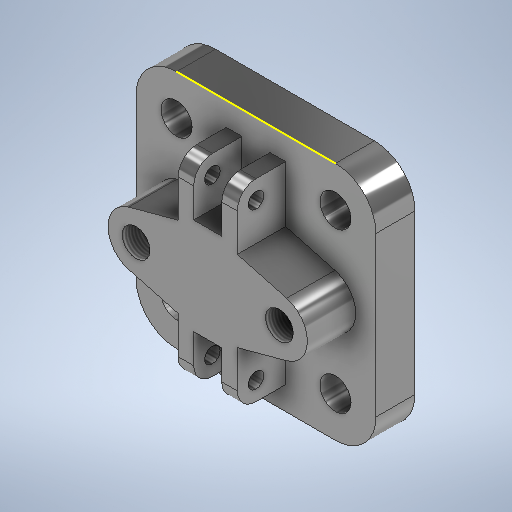
# Autodesk Inventor part: cad@74
Saved by Autodesk Inventor 2025.2 (Build 292293000, 293)
## iProperties
Created: 2025-04-27
Part Number: cad@74
Material: Generic
Document SubType Name: Modeling
Designer: spars
Density: 1 g/cm^3
Appearance: Chrome - Polished Black
Author: spars
Autodesk Inventor part; units mm, degrees
ref_plane "YZ Plane" through (0, 0, 0) normal (1, 0, 0) x (0, 1, 0)
ref_plane "XZ Plane" through (0, 0, 0) normal (0, 1, 0) x (-1, 0, 0)
ref_plane "XY Plane" through (0, 0, 0) normal (0, 0, 1) x (1, 0, 0)
sketch "Sketch1" plane through (0, 0, 0) normal (0, 0, 1) x (1, 0, 0)
  line L0 (-51, 77) -> (51, 77)
  line L1 (77, 51) -> (77, -51)
  line L2 (51, -77) -> (-51, -77)
  line L3 (-77, -51) -> (-77, 51)
  line L4 (-77, 77) -> (77, -77) construction
  line L5 (77, 77) -> (-77, -77) construction
  arc A0 (-51, 77) -> (-77, 51) centre (-51, 51) ccw
  arc A1 (-77, -51) -> (-51, -77) centre (-51, -51) ccw
  arc A2 (51, -77) -> (77, -51) centre (51, -51) ccw
  arc A3 (77, 51) -> (51, 77) centre (51, 51) ccw
  point P0 (0, 0)
  dimension "d0" = 154
  dimension "d1" = 154
  dimension "d2" = 26
  constraints: 12 end point, 8 point on circle, 8 point on line, 8 tangent, 4 centre point, 3 equal radius, 2 midpoint, 2 parallel, 1 horizontal, 1 perpendicular
  measures "d0" distance of L4.end L5.end
  measures "d1" distance of L5.start L4.end
  measures "d2" radius of A0
extrude "Extrusion1" add sketch "Sketch1" along normal blind 25
sketch "Sketch2" plane through (0, 0, 25) normal (0, 0, 1) x (1, 0, 0)
  arc A0 (-77, -51) -> (-51, -77) centre (-51, -51) ccw projected
  arc A1 (51, -77) -> (77, -51) centre (51, -51) ccw projected
  arc A2 (77, 51) -> (51, 77) centre (51, 51) ccw projected
  arc A3 (-51, 77) -> (-77, 51) centre (-51, 51) ccw projected
  point P0 (0, 0)
  constraints: 4 coincident
hole "Hole1" at (-51, -51, 25) at (51, -51, 25) at (51, 51, 25) at (-51, 51, 25) direction (0, 0, -1) diameter 20 end through all
sketch "Sketch3" plane through (0, 0, 0) normal (0, 0, -1) x (-1, 0, 0)
  circle A0 centre (0, 0) radius 56
  dimension "d12" = 112
  constraints: 1 centre point, 1 coincident
  measures "d12" diameter of A0
extrude "Extrusion2" add sketch "Sketch3" along normal blind 6
sketch "Sketch4" plane through (0, 0, 25) normal (0, 0, 1) x (1, 0, 0)
  line L0 (51, 77) -> (-51, 77) projected
sketch "Sketch5" plane through (0, 0, 25) normal (0, 0, 1) x (1, 0, 0)
  arc A0 (50.6713, -17.3833) -> (50.6713, 17.3833) centre (46, 0) ccw
  arc A1 (-50.6713, 17.3833) -> (-50.6713, -17.3833) centre (-46, 0) ccw
  line L0 (0, 31) -> (0, -31) construction
  line L1 (19, 62) -> (-19, -62) construction
  line L2 (-19, 62) -> (19, -62) construction
  line L3 (-9, 62) -> (-9, 31)
  line L4 (-9, 31) -> (9, 31)
  line L5 (9, 31) -> (9, 62)
  line L6 (-9, -62) -> (-9, -31)
  line L7 (-9, -31) -> (9, -31)
  line L8 (9, -31) -> (9, -62)
  line L9 (19, 62) -> (9, 62)
  line L10 (-9, 62) -> (-19, 62)
  line L11 (-19, -62) -> (-9, -62)
  line L12 (9, -62) -> (19, -62)
  line L13 (19, -62) -> (19, -25.8942)
  line L14 (19, 25.8942) -> (19, 62)
  line L15 (-19, 62) -> (-19, 25.8942)
  line L16 (-19, -25.8942) -> (-19, -62)
  line L17 (-19, 25.8942) -> (-50.6713, 17.3833)
  line L18 (-19, -25.8942) -> (-50.6713, -17.3833)
  line L19 (50.6713, -17.3833) -> (19, -25.8942)
  line L20 (50.6713, 17.3833) -> (19, 25.8942)
  point P0 (0, 0)
  dimension "d34" = 36
  dimension "d35" = 36
  dimension "d36" = 92
  dimension "d37" = 46
  dimension "d38" = 62
  dimension "d41" = 38
  dimension "d42" = 124
  dimension "d43" = 18
  dimension "d44" = 31
  dimension "d46" = 18
  dimension "d47" = 31
  constraints: 42 end point, 11 parallel, 4 perpendicular, 4 point on circle, 4 tangent, 3 midpoint, 2 centre point, 2 coincident, 2 horizontal, 1 horizontal alignment, 1 vertical
  measures "d34" diameter of A0
  measures "d35" diameter of A1
  measures "d36" distance of A1.centre A0.centre
  measures "d37" distance of point (0, 0) A1.centre
  measures "d38" distance of L0.start L0.end
  measures "d41" distance of L2.end L1.end
  measures "d42" distance of L1.end L2.start
  measures "d43" distance of L4.end L3.end
  measures "d44" distance of L3.end L3.start
  measures "d46" distance of L6.end L7.end
  measures "d47" distance of L6.start L6.end
extrude "Extrusion3" add sketch "Sketch5" along normal blind 31
sketch "Sketch6" plane through (0, 0, 56) normal (0, 0, 1) x (1, 0, 0)
  arc A0 (-50.6713, 17.3833) -> (-50.6713, -17.3833) centre (-46, 0) ccw projected
  arc A1 (50.6713, -17.3833) -> (50.6713, 17.3833) centre (46, 0) ccw projected
  point P0 (0, 0)
  constraints: 2 coincident
hole "Hole2" at (-46, 0, 56) at (46, 0, 56) direction (0, 0, -1) diameter 17.8349 depth 26 tip angle 118 thread size "M20x2" class "6H" standard "ISO Metric profile"
fillet "Fillet1" radius 12 4 edges at (-14, -62, 56) (14, -62, 56) (14, 62, 56) (-14, 62, 56)
sketch "Sketch7" plane through (-19, -62, 25) normal (-1, 0, 0) x (0, 0, 1)
  arc A0 (19, 0) -> (31, 12) centre (19, 12) ccw projected
  arc A1 (31, 112) -> (19, 124) centre (19, 112) ccw projected
  point P0 (-25, 62)
  constraints: 2 coincident
hole "Hole3" at (-19, -50, 44) at (-19, 50, 44) direction (1, 0, 0) diameter 10 end through all
equation "\"d37\" = 0.5 * d36"
body "Solid1"
